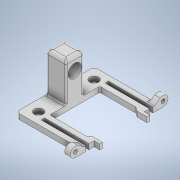
# Autodesk Inventor part: TopMount
Saved by Autodesk Inventor 2020 (Build 240168000, 168)
## iProperties
Created: 2020-07-01
Part Number: TopMount
Material: Generic
Document SubType Name: Modeling
Designer: lukep
Density: 1 g/cm^3
Appearance: Default
Author: lukep
Autodesk Inventor part; units mm, degrees
ref_plane "YZ Plane" through (0, 0, 0) normal (1, 0, 0) x (0, 1, 0)
ref_plane "XZ Plane" through (0, 0, 0) normal (0, 1, 0) x (-1, 0, 0)
ref_plane "XY Plane" through (0, 0, 0) normal (0, 0, 1) x (1, 0, 0)
sketch "Sketch1" plane through (0, 0, 0) normal (0, 1, 0) x (-1, 0, 0)
  line L0 (0, 0) -> (54.5, 0)
  line L1 (57.5, -3) -> (57.5, -67)
  line L2 (54.5, -70) -> (0, -70)
  circle A0 centre (47.5, -60) radius 4
  line L3 (57.5, -35) -> (0, -35) construction
  line L4 (0, -57.5) -> (38.5, -57.5)
  line L5 (40, -56) -> (40, -35)
  arc A1 (38.5, -57.5) -> (40, -56) centre (38.5, -56) ccw
  circle A2 centre (47.5, -10) radius 4
  line L6 (0, -12.5) -> (38.5, -12.5)
  line L7 (40, -14) -> (40, -35)
  arc A3 (40, -14) -> (38.5, -12.5) centre (38.5, -14) ccw
  line L8 (0, -70) -> (0, -57.5)
  line L9 (0, -12.5) -> (0, 0)
  arc A4 (54.5, -70) -> (57.5, -67) centre (54.5, -67) ccw
  arc A5 (57.5, -3) -> (54.5, 0) centre (54.5, -3) ccw
  point P0 (57.5, -70)
  point P1 (57.5, 0)
  dimension "d0" = 70
  dimension "d1" = 57.5
  dimension "d4" = 8
  dimension "d5" = 10
  dimension "d6" = 10
  dimension "d7" = 22.5
  dimension "d9" = 1.5
  dimension "d10" = 40
  dimension "d11" = 3
  constraints: 20 end point, 8 point on circle, 6 centre point, 6 tangent, 5 point on line, 5 symmetric about line, 4 perpendicular, 3 parallel, 1 equal radius, 1 horizontal, 1 midpoint, 2 other
  measures "d0" distance of point (57.5, 0) point (57.5, -70)
  measures "d1" distance of point (57.5, -70) L2.end
  measures "d4" diameter of A0
  measures "d5" distance from line of L2 A0.centre
  measures "d6" distance from line of L1 A0.centre
  measures "d7" distance between parallel lines of L3 L4
  measures "d9" radius of A1
  measures "d10" distance between parallel lines of L8 L5
  measures "d11" radius of A4
extrude "Extrusion1" add sketch "Sketch1" along normal blind 4.7625
sketch "Sketch5" plane through (0, 4.7625, 0) normal (0, 1, 0) x (1, 0, 0)
  line L0 (40, 7.75) -> (-40, 7.75)
  line L1 (-40, 7.75) -> (-40, 4.75)
  line L2 (-40, 4.75) -> (40, 4.75)
  line L3 (40, 4.75) -> (40, 7.75)
  line L4 (0, 0) -> (0, 12.5) projected
  line L5 (40, 7.75) -> (-40, 4.75) construction
  line L6 (-40, 7.75) -> (40, 4.75) construction
  line L7 (40, 65.25) -> (40, 62.25)
  line L8 (40, 62.25) -> (-40, 62.25)
  line L9 (-40, 62.25) -> (-40, 65.25)
  line L10 (-40, 65.25) -> (40, 65.25)
  line L11 (0, 57.5) -> (0, 70) projected
  line L12 (40, 65.25) -> (-40, 62.25) construction
  line L13 (40, 62.25) -> (-40, 65.25) construction
  line L14 (-40, 14) -> (-40, 56) projected
  point P0 (0, 6.25)
  point P1 (0, 63.75)
  point P2 (-40, 6.25)
  point P3 (-40, 63.75)
  point P4 (-40, 40.825)
  point P5 (0, 62.25)
  point P6 (0, 65.25)
  dimension "d45" = 0
  dimension "d46" = 3
  constraints: 24 end point, 8 midpoint, 4 parallel, 3 perpendicular, 1 collinear, 1 horizontal, 1 vertical alignment
  measures "d45" distance between parallel lines of L14 L1
  measures "d46" distance of L2.end L0.start
extrude "Extrusion5" cut sketch "Sketch5" against normal blind 25 contours L3 L2 L4 L0 | L4 L2 L1 L0 | L11 L8 L9 L10
sketch "Sketch6" plane through (0, 0, 0) normal (1, 0, 0) x (0, 0, -1)
  circle A0 centre (-4.5, 4.5) radius 4.5
  line L0 (0, 0) -> (4.75, 0) projected
  line L1 (0, 0) -> (0, 4.7625) projected
  line L2 (0, 0) -> (-4.5, 0)
  line L3 (3, 4.7625) -> (0, 4.7625) projected
  line L4 (3.1916, 4.7625) -> (-1.9948, 8.2382)
  line L5 (0, 0) -> (3.1916, 4.7625)
  circle A1 centre (-4.5, 4.5) radius 1.75
  line L6 (0, 0) -> (70.145, 0) construction
  line L7 (67, 0) -> (3, 0) construction
  line L8 (70.145, 0) -> (37.65, 0) construction
  line L9 (67, 4.7625) -> (3, 4.7625) construction
  line L10 (70, 0) -> (70, 4.7625) construction
  line L11 (70, 0) -> (70, 45.7679) construction
  line L12 (70, 45.7679) -> (0, 45.7679) construction
  line L13 (35, 45.7679) -> (35, 29.2895) construction
  circle A2 centre (74.5, 4.5) radius 4.5
  line L14 (70, 0) -> (65.25, 0)
  line L15 (70, 0) -> (70, 4.7625)
  line L16 (70, 0) -> (74.5, 0)
  line L17 (67, 4.7625) -> (70, 4.7625)
  line L18 (66.8084, 4.7625) -> (71.9948, 8.2382)
  line L19 (70, 0) -> (66.8084, 4.7625)
  circle A3 centre (74.5, 4.5) radius 1.75
  point P0 (37.65, 4.7625)
  dimension "d49" = 9
  dimension "d50" = 3.5
  constraints: 28 end point, 6 symmetric about line, 4 centre point, 4 point on circle, 4 tangent, 2 coincident, 2 perpendicular, 2 point on line, 2 vertical, 1 collinear, 1 horizontal, 1 midpoint, 2 other
  measures "d49" diameter of A0
  measures "d50" diameter of A1
extrude "Extrusion6" add sketch "Sketch6" against normal blind 5
fillet "Fillet6" radius 1.5875 5 edges at (-2.5, 4.7625, -3.1916) (-5, 2.3813, 0) (-5, 4.7625, -1.5958) (-5, 4.7625, -68.4042) (-5, 2.3813, -70)
sketch "Sketch7" plane through (-38.5, 0, -57.5) normal (0, 0, 1) x (1, 0, 0)
  line L0 (43.5, 0) -> (43.5, 4.7625)
  line L1 (43.5, 4.7625) -> (33.5, 4.7625)
  line L2 (33.5, 4.7625) -> (33.5, 0)
  line L3 (33.5, 0) -> (43.5, 0)
  line L4 (38.5, 0) -> (38.5, 4.7625) projected
  line L5 (43.5, 0) -> (33.5, 4.7625) construction
  line L6 (43.5, 4.7625) -> (33.5, 0) construction
  point P0 (38.5, 2.3813)
  dimension "d60" = 10
  constraints: 12 end point, 3 midpoint, 2 parallel, 1 perpendicular, 1 vertical
  measures "d60" distance of L0.end L1.end
extrude "Extrusion7" add sketch "Sketch7" along normal blind 2.5
sketch "Sketch8" plane through (0, 0, -12.5) normal (0, 0, -1) x (-1, 0, 0)
  line L0 (5, 0) -> (5, 4.7625)
  line L1 (5, 4.7625) -> (-5, 4.7625)
  line L2 (-5, 4.7625) -> (-5, 0)
  line L3 (-5, 0) -> (5, 0)
  line L4 (0, 0) -> (0, 4.7625) projected
  line L5 (5, 0) -> (-5, 4.7625) construction
  line L6 (5, 4.7625) -> (-5, 0) construction
  point P0 (0, 2.3813)
  dimension "d63" = 10
  constraints: 12 end point, 3 midpoint, 3 parallel, 1 perpendicular
  measures "d63" distance of L1.end L0.end
extrude "Extrusion8" add sketch "Sketch8" along normal blind 2.5
fillet "Fillet7" radius 3.175 4 edges at (-5, 2.3813, -12.5) (-5, 2.3813, -15) (-5, 2.3812, -57.5) (-5, 2.3812, -55)
sketch "Sketch9" plane through (0, 4.7625, 0) normal (0, 1, 0) x (1, 0, 0)
  line L0 (-40, 14) -> (-40, 56) projected
  line L1 (-57.5, 67) -> (-57.5, 3) projected
  line L2 (-57.5, 29.926) -> (-57.5, 43)
  line L3 (-57.5, 43) -> (-40, 43)
  line L4 (-40, 43) -> (-40, 26.926)
  line L5 (-54.5, 0) -> (-6.5875, 0) projected
  line L6 (-40, 43) -> (-40, 27)
  line L7 (-40, 27) -> (-57.5, 27)
  line L8 (-57.5, 27) -> (-57.5, 43)
  point P0 (0, 0)
  point P1 (-40, 43)
  dimension "d88" = 16
  dimension "d89" = 27
  constraints: 12 end point, 3 point on line, 2 parallel
  measures "d88" distance between parallel lines of L7 L3
  measures "d89" distance between parallel lines of L5 L7
extrude "Extrusion9" add sketch "Sketch9" along normal blind 35
fillet "Fillet9" radius 1.5 5 edges at (-40, 22.2625, -43) (-40, 22.2625, -27) (-57.5, 22.2625, -27) (-48.75, 4.7625, -27) (-48.75, 4.7625, -43)
sketch "Sketch11" plane through (-40, 0, -14) normal (1, 0, 0) x (0, 0, -1)
  circle A0 centre (21, 28) radius 6
  line L0 (0, 0) -> (42, 0) projected
  point P0 (-14, 0)
  dimension "d90" = 12
  dimension "d91" = 28
  constraints: 1 centre point
  measures "d90" diameter of A0
  measures "d91" distance from line of L0 A0.centre
extrude "Extrusion11" cut sketch "Sketch11" against normal blind 35
fillet "Fillet10" radius 3.175 7 edges at (-40.4393, 39.7625, -27.4393) (-40, 39.7625, -35) (-40.4393, 39.7625, -42.5607) (-49.5, 39.7625, -43) (-57.0607, 39.7625, -27.4393) (-57.5, 39.7625, -35.75) (-48.75, 39.7625, -27)
body "Solid1"
